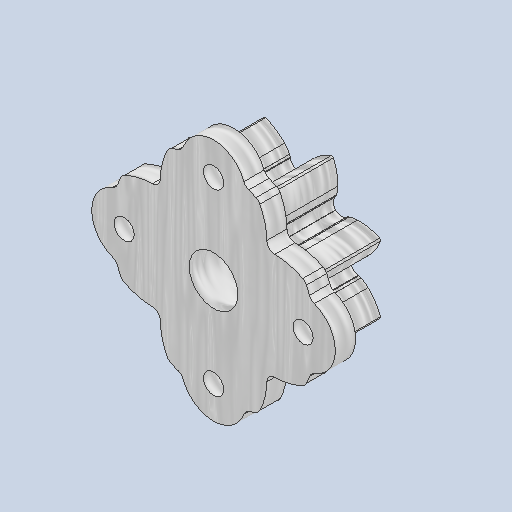
# Autodesk Inventor part: アーム 2段目ギア 小ギア 8
Saved by Autodesk Inventor 2023 (Build 270158030, 158C)
## iProperties
Created: 2020-05-02
Part Number: アーム 2段目ギア 小ギア 8
Material: アルミニウム 7075
Document SubType Name: Modeling
Designer: mozar
Density: 2.81 g/cm^3
Appearance: サテン - ブラシ仕上げ 重厚
Author: mozar
Autodesk Inventor part; units mm, degrees
ref_plane "YZ Plane" through (0, 0, 0) normal (1, 0, 0) x (0, 1, 0)
ref_plane "XZ Plane" through (0, 0, 0) normal (0, 1, 0) x (-1, 0, 0)
ref_plane "XY Plane" through (0, 0, 0) normal (0, 0, 1) x (1, 0, 0)
sketch "スケッチ1" plane through (0, 0, 0) normal (0, 0, 1) x (1, 0, 0)
  arc A0 (149.6102, 112.7227) -> (149.5189, 112.4482) centre (150.664, 112.2197) ccw
  arc A1 (150.2091, 113.6063) -> (149.6102, 112.7227) centre (152.6236, 111.3248) ccw
  arc A2 (152.5503, 115.1567) -> (150.2091, 113.6063) centre (154.7206, 109.3368) ccw
  arc A3 (143.8242, 111.2458) -> (143.9538, 110.9871) centre (144.9251, 111.6353) ccw
  arc A4 (143.623, 112.2941) -> (143.8242, 111.2458) centre (146.9435, 112.3881) ccw
  arc A5 (144.1821, 115.0459) -> (143.623, 112.2941) centre (149.832, 112.4652) ccw
  arc A6 (140.7773, 106.1102) -> (141.0518, 106.0189) centre (141.2803, 107.164) ccw
  arc A7 (139.8937, 106.7091) -> (140.7773, 106.1102) centre (142.1752, 109.1236) ccw
  arc A8 (138.3433, 109.0503) -> (139.8937, 106.7091) centre (144.1632, 111.2206) ccw
  arc A9 (142.2542, 100.3242) -> (142.5129, 100.4538) centre (141.8647, 101.4251) ccw
  arc A10 (141.2059, 100.123) -> (142.2542, 100.3242) centre (141.1119, 103.4435) ccw
  arc A11 (138.4541, 100.6821) -> (141.2059, 100.123) centre (141.0348, 106.332) ccw
  arc A12 (147.3898, 97.2773) -> (147.4811, 97.5518) centre (146.336, 97.7803) ccw
  arc A13 (146.7909, 96.3937) -> (147.3898, 97.2773) centre (144.3764, 98.6752) ccw
  arc A14 (144.4497, 94.8433) -> (146.7909, 96.3937) centre (142.2794, 100.6632) ccw
  arc A15 (153.1758, 98.7542) -> (153.0462, 99.0129) centre (152.0749, 98.3647) ccw
  arc A16 (153.377, 97.7059) -> (153.1758, 98.7542) centre (150.0565, 97.6119) ccw
  arc A17 (152.8179, 94.9541) -> (153.377, 97.7059) centre (147.168, 97.5348) ccw
  arc A18 (156.2227, 103.8898) -> (155.9482, 103.9811) centre (155.7197, 102.836) ccw
  arc A19 (157.1063, 103.2909) -> (156.2227, 103.8898) centre (154.8248, 100.8764) ccw
  arc A20 (158.6567, 100.9497) -> (157.1063, 103.2909) centre (152.8368, 98.7794) ccw
  arc A21 (154.7458, 109.6758) -> (154.4871, 109.5462) centre (155.1353, 108.5749) ccw
  arc A22 (155.7941, 109.877) -> (154.7458, 109.6758) centre (155.8881, 106.5565) ccw
  arc A23 (158.5459, 109.3179) -> (155.7941, 109.877) centre (155.9652, 103.668) ccw
  arc A24 (147.4811, 112.4482) -> (147.3898, 112.7227) centre (146.336, 112.2197) ccw
  arc A25 (147.3898, 112.7227) -> (146.7909, 113.6063) centre (144.3764, 111.3248) ccw
  arc A26 (146.7909, 113.6063) -> (144.4497, 115.1567) centre (142.2794, 109.3368) ccw
  arc A27 (142.5129, 109.5462) -> (142.2542, 109.6758) centre (141.8647, 108.5749) ccw
  arc A28 (142.2542, 109.6758) -> (141.2059, 109.877) centre (141.1119, 106.5565) ccw
  arc A29 (141.2059, 109.877) -> (138.4541, 109.3179) centre (141.0348, 103.668) ccw
  arc A30 (141.0518, 103.9811) -> (140.7773, 103.8898) centre (141.2803, 102.836) ccw
  arc A31 (140.7773, 103.8898) -> (139.8937, 103.2909) centre (142.1752, 100.8764) ccw
  arc A32 (139.8937, 103.2909) -> (138.3433, 100.9497) centre (144.1632, 98.7794) ccw
  arc A33 (143.9538, 99.0129) -> (143.8242, 98.7542) centre (144.9251, 98.3647) ccw
  arc A34 (143.8242, 98.7542) -> (143.623, 97.7059) centre (146.9435, 97.6119) ccw
  arc A35 (143.623, 97.7059) -> (144.1821, 94.9541) centre (149.832, 97.5348) ccw
  arc A36 (149.5189, 97.5518) -> (149.6102, 97.2773) centre (150.664, 97.7803) ccw
  arc A37 (149.6102, 97.2773) -> (150.2091, 96.3937) centre (152.6236, 98.6752) ccw
  arc A38 (150.2091, 96.3937) -> (152.5503, 94.8433) centre (154.7206, 100.6632) ccw
  arc A39 (154.4871, 100.4538) -> (154.7458, 100.3242) centre (155.1353, 101.4251) ccw
  arc A40 (154.7458, 100.3242) -> (155.7941, 100.123) centre (155.8881, 103.4435) ccw
  arc A41 (155.7941, 100.123) -> (158.5459, 100.6821) centre (155.9652, 106.332) ccw
  arc A42 (155.9482, 106.0189) -> (156.2227, 106.1102) centre (155.7197, 107.164) ccw
  arc A43 (156.2227, 106.1102) -> (157.1063, 106.7091) centre (154.8248, 109.1236) ccw
  arc A44 (157.1063, 106.7091) -> (158.6567, 109.0503) centre (152.8368, 111.2206) ccw
  arc A45 (153.0462, 110.9871) -> (153.1758, 111.2458) centre (152.0749, 111.6353) ccw
  arc A46 (153.1758, 111.2458) -> (153.377, 112.2941) centre (150.0565, 112.3881) ccw
  arc A47 (153.377, 112.2941) -> (152.8179, 115.0459) centre (147.168, 112.4652) ccw
  arc A48 (149.3809, 111.44) -> (147.6191, 111.44) centre (148.5, 105) ccw
  arc A49 (144.5691, 110.1767) -> (143.3233, 108.9309) centre (148.5, 105) ccw
  arc A50 (142.06, 105.8809) -> (142.06, 104.1191) centre (148.5, 105) ccw
  arc A51 (143.3233, 101.0691) -> (144.5691, 99.8233) centre (148.5, 105) ccw
  arc A52 (147.6191, 98.56) -> (149.3809, 98.56) centre (148.5, 105) ccw
  arc A53 (152.4309, 99.8233) -> (153.6767, 101.0691) centre (148.5, 105) ccw
  arc A54 (154.94, 104.1191) -> (154.94, 105.8809) centre (148.5, 105) ccw
  arc A55 (153.6767, 108.9309) -> (152.4309, 110.1767) centre (148.5, 105) ccw
  arc A56 (144.4497, 115.1567) -> (144.1821, 115.0459) centre (148.5, 105) ccw
  arc A57 (138.4541, 109.3179) -> (138.3433, 109.0503) centre (148.5, 105) ccw
  arc A58 (138.3433, 100.9497) -> (138.4541, 100.6821) centre (148.5, 105) ccw
  arc A59 (144.1821, 94.9541) -> (144.4497, 94.8433) centre (148.5, 105) ccw
  arc A60 (152.5503, 94.8433) -> (152.8179, 94.9541) centre (148.5, 105) ccw
  arc A61 (158.5459, 100.6821) -> (158.6567, 100.9497) centre (148.5, 105) ccw
  arc A62 (158.6567, 109.0503) -> (158.5459, 109.3179) centre (148.5, 105) ccw
  arc A63 (152.8179, 115.0459) -> (152.5503, 115.1567) centre (148.5, 105) ccw
  line L0 (149.3809, 111.44) -> (149.5189, 112.4482)
  line L1 (144.5691, 110.1767) -> (143.9538, 110.9871)
  line L2 (142.06, 105.8809) -> (141.0518, 106.0189)
  line L3 (143.3233, 101.0691) -> (142.5129, 100.4538)
  line L4 (147.6191, 98.56) -> (147.4811, 97.5518)
  line L5 (152.4309, 99.8233) -> (153.0462, 99.0129)
  line L6 (154.94, 104.1191) -> (155.9482, 103.9811)
  line L7 (153.6767, 108.9309) -> (154.4871, 109.5462)
  line L8 (147.6191, 111.44) -> (147.4811, 112.4482)
  line L9 (143.3233, 108.9309) -> (142.5129, 109.5462)
  line L10 (142.06, 104.1191) -> (141.0518, 103.9811)
  line L11 (144.5691, 99.8233) -> (143.9538, 99.0129)
  line L12 (149.3809, 98.56) -> (149.5189, 97.5518)
  line L13 (153.6767, 101.0691) -> (154.4871, 100.4538)
  line L14 (154.94, 105.8809) -> (155.9482, 106.0189)
  line L15 (152.4309, 110.1767) -> (153.0462, 110.9871)
  line L16 (135.5655, 105) -> (161.4345, 105)
  line L17 (148.5, 92.0655) -> (148.5, 117.9345)
  line L18 (179.4346, 115.9346) -> (249.4346, 115.9346)
  line L19 (179.4346, 107.9346) -> (249.4346, 107.9346)
  line L20 (179.4346, 99.9346) -> (249.4346, 99.9346)
  line L21 (179.4346, 91.9346) -> (249.4346, 91.9346)
  line L22 (179.4346, 83.9346) -> (249.4346, 83.9346)
  line L23 (179.4346, 75.9346) -> (249.4346, 75.9346)
  line L24 (179.4346, 67.9346) -> (249.4346, 67.9346)
  line L25 (179.4346, 59.9346) -> (249.4346, 59.9346)
  line L26 (179.4346, 51.9346) -> (249.4346, 51.9346)
  line L27 (179.4346, 43.9346) -> (249.4346, 43.9346)
  line L28 (179.4346, 35.9346) -> (249.4346, 35.9346)
  line L29 (179.4346, 27.9346) -> (249.4346, 27.9346)
  line L30 (179.4346, 19.9346) -> (249.4346, 19.9346)
  line L31 (179.4346, 115.9346) -> (179.4346, 19.9346)
  line L32 (249.4346, 115.9346) -> (249.4346, 19.9346)
  line L33 (214.4346, 107.9346) -> (214.4346, 19.9346)
  point P0 (0, 0)
  point P1 (185.4346, 109.9346)
  point P2 (187.9346, 101.9346)
  point P3 (187.9346, 93.9346)
  point P4 (185.4346, 85.9346)
  point P5 (187.9346, 77.9346)
  point P6 (182.9346, 69.9346)
  point P7 (185.4346, 61.9346)
  point P8 (185.4346, 53.9346)
  point P9 (185.4346, 45.9346)
  point P10 (187.9346, 37.9346)
  point P11 (187.9346, 29.9346)
  point P12 (185.4346, 21.9346)
  point P13 (215.4346, 101.9346)
  point P14 (231.6846, 93.9346)
  point P15 (231.6846, 85.9346)
  point P16 (227.9346, 77.9346)
  point P17 (230.4346, 69.9346)
  point P18 (224.1846, 61.9346)
  point P19 (224.1846, 53.9346)
  point P20 (230.4346, 45.9346)
  point P21 (225.4346, 37.9346)
  point P22 (232.9346, 29.9346)
  point P23 (232.9346, 21.9346)
  point P24 (149.5, 131.4345)
  point P25 (149.5, 125.4345)
  point P26 (166.75, 131.4345)
  point P27 (168.875, 125.4345)
  constraints: 128 point on circle, 64 centre point, 64 end point, 2 midpoint, 1 horizontal, 1 vertical, 268 other
extrude "押し出し1" add sketch "スケッチ1" against normal blind 8 contours A1 A2 A63 A47 A46 A45 L15 A55 L7 A21 A22 A23 A62 A44 A43 A42 L14 A54 L16 L17 A48 L0 A0 | L17 L16 A50 L2 A6 A7 A8 A57 A29 A28 A27 L9 A49 L1 A3 A4 A5 A56 A26 A25 A24 L8 A48 | L17 A52 L4 A12 A13 A14 A59 A35 A34 A33 L11 A51 L3 A9 A10 A11 A58 A32 A31 A30 L10 A50 L16 | L16 A54 L6 A18 A19 A20 A61 A41 A40 A39 L13 A53 L5 A15 A16 A17 A60 A38 A37 A36 L12 A52 L17
fillet "フィレット1" radius 1 16 edges at (142.06, 105.8809, -4) (143.3233, 108.9309, -4) (144.5691, 110.1767, -4) (147.6191, 111.44, -4) (149.3809, 111.44, -4) (152.4309, 110.1767, -4) (153.6767, 108.9309, -4) (154.94, 105.8809, -4) (154.94, 104.1191, -4) (153.6767, 101.0691, -4) (152.4309, 99.8233, -4) (149.3809, 98.56, -4) (147.6191, 98.56, -4) (144.5691, 99.8233, -4) (143.3233, 101.0691, -4) (142.06, 104.1191, -4)
sketch "スケッチ2" plane through (0, 0, 0) normal (0, 0, 1) x (1, 0, 0)
  arc A0 (153.1771, 111.2494) -> (153.1747, 111.2428) centre (154.1165, 110.9066) ccw projected
  arc A1 (153.0462, 110.9871) -> (153.1747, 111.2428) centre (152.0749, 111.6353) ccw projected
  line L0 (153.0462, 110.9871) -> (152.9951, 110.9198) projected
  arc A2 (152.9951, 110.9198) -> (153.086, 109.6064) centre (153.7915, 110.315) ccw projected
  arc A3 (153.1064, 109.586) -> (153.086, 109.6064) centre (148.5, 105) ccw projected
  arc A4 (153.1064, 109.586) -> (154.4198, 109.4951) centre (153.815, 110.2915) ccw projected
  line L1 (154.4198, 109.4951) -> (154.4871, 109.5462) projected
  arc A5 (154.7428, 109.6747) -> (154.4871, 109.5462) centre (155.1353, 108.5749) ccw projected
  arc A6 (154.7428, 109.6747) -> (154.7494, 109.6771) centre (154.4066, 110.6165) ccw projected
  arc A7 (155.7941, 109.877) -> (154.7494, 109.6771) centre (155.8881, 106.5565) ccw projected
  arc A8 (158.5459, 109.3179) -> (155.7941, 109.877) centre (155.9652, 103.668) ccw projected
  arc A9 (158.6567, 109.0503) -> (158.5459, 109.3179) centre (148.5, 105) ccw projected
  arc A10 (157.1063, 106.7091) -> (158.6567, 109.0503) centre (152.8368, 111.2206) ccw projected
  arc A11 (156.2262, 106.1118) -> (157.1063, 106.7091) centre (154.8248, 109.1236) ccw projected
  arc A12 (156.2262, 106.1118) -> (156.2198, 106.1088) centre (156.6481, 105.2052) ccw projected
  arc A13 (155.9482, 106.0189) -> (156.2198, 106.1088) centre (155.7197, 107.164) ccw projected
  line L2 (155.9482, 106.0189) -> (155.8645, 106.0074) projected
  arc A14 (155.8645, 106.0074) -> (155, 105.0144) centre (156, 105.0166) ccw projected
  arc A15 (155, 104.9856) -> (155, 105.0144) centre (148.5, 105) ccw projected
  arc A16 (155, 104.9856) -> (155.8645, 103.9926) centre (156, 104.9834) ccw projected
  line L3 (155.8645, 103.9926) -> (155.9482, 103.9811) projected
  arc A17 (156.2198, 103.8912) -> (155.9482, 103.9811) centre (155.7197, 102.836) ccw projected
  arc A18 (156.2198, 103.8912) -> (156.2262, 103.8882) centre (156.6481, 104.7948) ccw projected
  arc A19 (157.1063, 103.2909) -> (156.2262, 103.8882) centre (154.8248, 100.8764) ccw projected
  arc A20 (158.6567, 100.9497) -> (157.1063, 103.2909) centre (152.8368, 98.7794) ccw projected
  arc A21 (158.5459, 100.6821) -> (158.6567, 100.9497) centre (148.5, 105) ccw projected
  arc A22 (155.7941, 100.123) -> (158.5459, 100.6821) centre (155.9652, 106.332) ccw projected
  arc A23 (154.7494, 100.3229) -> (155.7941, 100.123) centre (155.8881, 103.4435) ccw projected
  arc A24 (154.7494, 100.3229) -> (154.7428, 100.3253) centre (154.4066, 99.3835) ccw projected
  arc A25 (154.4871, 100.4538) -> (154.7428, 100.3253) centre (155.1353, 101.4251) ccw projected
  line L4 (154.4871, 100.4538) -> (154.4198, 100.5049) projected
  arc A26 (154.4198, 100.5049) -> (153.1064, 100.414) centre (153.815, 99.7085) ccw projected
  arc A27 (153.086, 100.3936) -> (153.1064, 100.414) centre (148.5, 105) ccw projected
  arc A28 (153.086, 100.3936) -> (152.9951, 99.0802) centre (153.7915, 99.685) ccw projected
  line L5 (152.9951, 99.0802) -> (153.0462, 99.0129) projected
  arc A29 (153.1747, 98.7572) -> (153.0462, 99.0129) centre (152.0749, 98.3647) ccw projected
  arc A30 (153.1747, 98.7572) -> (153.1771, 98.7506) centre (154.1165, 99.0934) ccw projected
  arc A31 (153.377, 97.7059) -> (153.1771, 98.7506) centre (150.0565, 97.6119) ccw projected
  arc A32 (152.8179, 94.9541) -> (153.377, 97.7059) centre (147.168, 97.5348) ccw projected
  arc A33 (152.5503, 94.8433) -> (152.8179, 94.9541) centre (148.5, 105) ccw projected
  arc A34 (150.2091, 96.3937) -> (152.5503, 94.8433) centre (154.7206, 100.6632) ccw projected
  arc A35 (149.6118, 97.2738) -> (150.2091, 96.3937) centre (152.6236, 98.6752) ccw projected
  arc A36 (149.6118, 97.2738) -> (149.6088, 97.2802) centre (148.7052, 96.8519) ccw projected
  arc A37 (149.5189, 97.5518) -> (149.6088, 97.2802) centre (150.664, 97.7803) ccw projected
  line L6 (149.5189, 97.5518) -> (149.5074, 97.6355) projected
  arc A38 (149.5074, 97.6355) -> (148.5144, 98.5) centre (148.5166, 97.5) ccw projected
  arc A39 (148.4856, 98.5) -> (148.5144, 98.5) centre (148.5, 105) ccw projected
  arc A40 (148.4856, 98.5) -> (147.4926, 97.6355) centre (148.4834, 97.5) ccw projected
  line L7 (147.4926, 97.6355) -> (147.4811, 97.5518) projected
  arc A41 (147.3912, 97.2802) -> (147.4811, 97.5518) centre (146.336, 97.7803) ccw projected
  arc A42 (147.3912, 97.2802) -> (147.3882, 97.2738) centre (148.2948, 96.8519) ccw projected
  arc A43 (146.7909, 96.3937) -> (147.3882, 97.2738) centre (144.3764, 98.6752) ccw projected
  arc A44 (144.4497, 94.8433) -> (146.7909, 96.3937) centre (142.2794, 100.6632) ccw projected
  arc A45 (144.1821, 94.9541) -> (144.4497, 94.8433) centre (148.5, 105) ccw projected
  arc A46 (143.623, 97.7059) -> (144.1821, 94.9541) centre (149.832, 97.5348) ccw projected
  arc A47 (143.8229, 98.7506) -> (143.623, 97.7059) centre (146.9435, 97.6119) ccw projected
  arc A48 (143.8229, 98.7506) -> (143.8253, 98.7572) centre (142.8835, 99.0934) ccw projected
  arc A49 (143.9538, 99.0129) -> (143.8253, 98.7572) centre (144.9251, 98.3647) ccw projected
  line L8 (143.9538, 99.0129) -> (144.0049, 99.0802) projected
  arc A50 (144.0049, 99.0802) -> (143.914, 100.3936) centre (143.2085, 99.685) ccw projected
  arc A51 (143.8936, 100.414) -> (143.914, 100.3936) centre (148.5, 105) ccw projected
  arc A52 (143.8936, 100.414) -> (142.5802, 100.5049) centre (143.185, 99.7085) ccw projected
  line L9 (142.5802, 100.5049) -> (142.5129, 100.4538) projected
  arc A53 (142.2572, 100.3253) -> (142.5129, 100.4538) centre (141.8647, 101.4251) ccw projected
  arc A54 (142.2572, 100.3253) -> (142.2506, 100.3229) centre (142.5934, 99.3835) ccw projected
  arc A55 (141.2059, 100.123) -> (142.2506, 100.3229) centre (141.1119, 103.4435) ccw projected
  arc A56 (138.4541, 100.6821) -> (141.2059, 100.123) centre (141.0348, 106.332) ccw projected
  arc A57 (138.3433, 100.9497) -> (138.4541, 100.6821) centre (148.5, 105) ccw projected
  arc A58 (139.8937, 103.2909) -> (138.3433, 100.9497) centre (144.1632, 98.7794) ccw projected
  arc A59 (140.7738, 103.8882) -> (139.8937, 103.2909) centre (142.1752, 100.8764) ccw projected
  arc A60 (140.7738, 103.8882) -> (140.7802, 103.8912) centre (140.3519, 104.7948) ccw projected
  arc A61 (141.0518, 103.9811) -> (140.7802, 103.8912) centre (141.2803, 102.836) ccw projected
  line L10 (141.0518, 103.9811) -> (141.1355, 103.9926) projected
  arc A62 (141.1355, 103.9926) -> (142, 104.9856) centre (141, 104.9834) ccw projected
  arc A63 (142, 105.0144) -> (142, 104.9856) centre (148.5, 105) ccw projected
  arc A64 (142, 105.0144) -> (141.1355, 106.0074) centre (141, 105.0166) ccw projected
  line L11 (141.1355, 106.0074) -> (141.0518, 106.0189) projected
  arc A65 (140.7802, 106.1088) -> (141.0518, 106.0189) centre (141.2803, 107.164) ccw projected
  arc A66 (140.7802, 106.1088) -> (140.7738, 106.1118) centre (140.3519, 105.2052) ccw projected
  arc A67 (139.8937, 106.7091) -> (140.7738, 106.1118) centre (142.1752, 109.1236) ccw projected
  arc A68 (138.3433, 109.0503) -> (139.8937, 106.7091) centre (144.1632, 111.2206) ccw projected
  arc A69 (138.4541, 109.3179) -> (138.3433, 109.0503) centre (148.5, 105) ccw projected
  arc A70 (141.2059, 109.877) -> (138.4541, 109.3179) centre (141.0348, 103.668) ccw projected
  arc A71 (142.2506, 109.6771) -> (141.2059, 109.877) centre (141.1119, 106.5565) ccw projected
  arc A72 (142.2506, 109.6771) -> (142.2572, 109.6747) centre (142.5934, 110.6165) ccw projected
  arc A73 (142.5129, 109.5462) -> (142.2572, 109.6747) centre (141.8647, 108.5749) ccw projected
  line L12 (142.5129, 109.5462) -> (142.5802, 109.4951) projected
  arc A74 (142.5802, 109.4951) -> (143.8936, 109.586) centre (143.185, 110.2915) ccw projected
  arc A75 (143.914, 109.6064) -> (143.8936, 109.586) centre (148.5, 105) ccw projected
  arc A76 (143.914, 109.6064) -> (144.0049, 110.9198) centre (143.2085, 110.315) ccw projected
  line L13 (144.0049, 110.9198) -> (143.9538, 110.9871) projected
  arc A77 (143.8253, 111.2428) -> (143.9538, 110.9871) centre (144.9251, 111.6353) ccw projected
  arc A78 (143.8253, 111.2428) -> (143.8229, 111.2494) centre (142.8835, 110.9066) ccw projected
  arc A79 (143.623, 112.2941) -> (143.8229, 111.2494) centre (146.9435, 112.3881) ccw projected
  arc A80 (144.1821, 115.0459) -> (143.623, 112.2941) centre (149.832, 112.4652) ccw projected
  arc A81 (144.4497, 115.1567) -> (144.1821, 115.0459) centre (148.5, 105) ccw projected
  arc A82 (146.7909, 113.6063) -> (144.4497, 115.1567) centre (142.2794, 109.3368) ccw projected
  arc A83 (147.3882, 112.7262) -> (146.7909, 113.6063) centre (144.3764, 111.3248) ccw projected
  arc A84 (147.3882, 112.7262) -> (147.3912, 112.7198) centre (148.2948, 113.1481) ccw projected
  arc A85 (147.4811, 112.4482) -> (147.3912, 112.7198) centre (146.336, 112.2197) ccw projected
  line L14 (147.4811, 112.4482) -> (147.4926, 112.3645) projected
  arc A86 (147.4926, 112.3645) -> (148.4856, 111.5) centre (148.4834, 112.5) ccw projected
  arc A87 (148.5144, 111.5) -> (148.4856, 111.5) centre (148.5, 105) ccw projected
  arc A88 (148.5144, 111.5) -> (149.5074, 112.3645) centre (148.5166, 112.5) ccw projected
  line L15 (149.5074, 112.3645) -> (149.5189, 112.4482) projected
  arc A89 (149.6088, 112.7198) -> (149.5189, 112.4482) centre (150.664, 112.2197) ccw projected
  arc A90 (149.6088, 112.7198) -> (149.6118, 112.7262) centre (148.7052, 113.1481) ccw projected
  arc A91 (150.2091, 113.6063) -> (149.6118, 112.7262) centre (152.6236, 111.3248) ccw projected
  arc A92 (152.5503, 115.1567) -> (150.2091, 113.6063) centre (154.7206, 109.3368) ccw projected
  arc A93 (152.8179, 115.0459) -> (152.5503, 115.1567) centre (148.5, 105) ccw projected
  arc A94 (153.377, 112.2941) -> (152.8179, 115.0459) centre (147.168, 112.4652) ccw projected
  arc A95 (153.1771, 111.2494) -> (153.377, 112.2941) centre (150.0565, 112.3881) ccw projected
  arc A96 (148.0715, 113.4456) -> (149.5921, 109.5599) centre (150.664, 112.2197) ccw
  line L16 (149.5921, 109.5599) -> (149.16, 112.7186)
  arc A97 (149.16, 112.7186) -> (148.9285, 113.4456) centre (146.336, 112.2197) ccw
  arc A98 (148.9285, 113.4456) -> (148.0209, 114.7797) centre (144.3764, 111.3248) ccw
  arc A99 (148.0209, 114.7797) -> (144.4127, 116.9552) centre (142.2794, 109.3368) ccw
  arc A100 (144.4127, 116.9552) -> (142.9366, 116.3437) centre (148.5, 105) ccw
  arc A101 (142.9366, 116.3437) -> (141.9234, 112.2541) centre (149.832, 112.4652) ccw
  arc A102 (141.9234, 112.2541) -> (142.2251, 110.6689) centre (146.9435, 112.3881) ccw
  arc A103 (142.2251, 110.6689) -> (142.5754, 109.9912) centre (144.9251, 111.6353) ccw
  line L17 (142.5754, 109.9912) -> (144.5035, 107.4521)
  arc A104 (144.5035, 107.4521) -> (142.8311, 111.2749) centre (141.8647, 108.5749) ccw
  arc A105 (142.8311, 111.2749) -> (141.2459, 111.5766) centre (141.1119, 106.5565) ccw
  arc A106 (141.2459, 111.5766) -> (137.1563, 110.5634) centre (141.0348, 103.668) ccw
  arc A107 (137.1563, 110.5634) -> (136.5448, 109.0873) centre (148.5, 105) ccw
  arc A108 (136.5448, 109.0873) -> (138.7203, 105.4791) centre (144.1632, 111.2206) ccw
  arc A109 (138.7203, 105.4791) -> (140.0544, 104.5715) centre (142.1752, 109.1236) ccw
  arc A110 (140.0544, 104.5715) -> (143.9401, 106.0921) centre (141.2803, 107.164) ccw
  line L18 (143.9401, 106.0921) -> (140.7814, 105.66)
  arc A111 (140.7814, 105.66) -> (140.0544, 105.4285) centre (141.2803, 102.836) ccw
  arc A112 (140.0544, 105.4285) -> (138.7203, 104.5209) centre (142.1752, 100.8764) ccw
  arc A113 (138.7203, 104.5209) -> (136.5448, 100.9127) centre (144.1632, 98.7794) ccw
  arc A114 (136.5448, 100.9127) -> (137.1563, 99.4366) centre (148.5, 105) ccw
  arc A115 (137.1563, 99.4366) -> (141.2459, 98.4234) centre (141.0348, 106.332) ccw
  arc A116 (141.2459, 98.4234) -> (142.8311, 98.7251) centre (141.1119, 103.4435) ccw
  arc A117 (142.8311, 98.7251) -> (143.5088, 99.0754) centre (141.8647, 101.4251) ccw
  line L19 (143.5088, 99.0754) -> (146.0479, 101.0035)
  arc A118 (146.0479, 101.0035) -> (142.2251, 99.3311) centre (144.9251, 98.3647) ccw
  arc A119 (142.2251, 99.3311) -> (141.9234, 97.7459) centre (146.9435, 97.6119) ccw
  arc A120 (141.9234, 97.7459) -> (142.9366, 93.6563) centre (149.832, 97.5348) ccw
  arc A121 (142.9366, 93.6563) -> (144.4127, 93.0448) centre (148.5, 105) ccw
  arc A122 (144.4127, 93.0448) -> (148.0209, 95.2203) centre (142.2794, 100.6632) ccw
  arc A123 (148.0209, 95.2203) -> (148.9285, 96.5544) centre (144.3764, 98.6752) ccw
  arc A124 (148.9285, 96.5544) -> (147.4079, 100.4401) centre (146.336, 97.7803) ccw
  line L20 (147.4079, 100.4401) -> (147.84, 97.2814)
  arc A125 (147.84, 97.2814) -> (148.0715, 96.5544) centre (150.664, 97.7803) ccw
  arc A126 (148.0715, 96.5544) -> (148.9791, 95.2203) centre (152.6236, 98.6752) ccw
  arc A127 (148.9791, 95.2203) -> (152.5873, 93.0448) centre (154.7206, 100.6632) ccw
  arc A128 (152.5873, 93.0448) -> (154.0634, 93.6563) centre (148.5, 105) ccw
  arc A129 (154.0634, 93.6563) -> (155.0766, 97.7459) centre (147.168, 97.5348) ccw
  arc A130 (155.0766, 97.7459) -> (154.7749, 99.3311) centre (150.0565, 97.6119) ccw
  arc A131 (154.7749, 99.3311) -> (154.4246, 100.0088) centre (152.0749, 98.3647) ccw
  line L21 (154.4246, 100.0088) -> (152.4965, 102.5479)
  arc A132 (152.4965, 102.5479) -> (154.1689, 98.7251) centre (155.1353, 101.4251) ccw
  arc A133 (154.1689, 98.7251) -> (155.7541, 98.4234) centre (155.8881, 103.4435) ccw
  arc A134 (155.7541, 98.4234) -> (159.8437, 99.4366) centre (155.9652, 106.332) ccw
  arc A135 (159.8437, 99.4366) -> (160.4552, 100.9127) centre (148.5, 105) ccw
  arc A136 (160.4552, 100.9127) -> (158.2797, 104.5209) centre (152.8368, 98.7794) ccw
  arc A137 (158.2797, 104.5209) -> (156.9456, 105.4285) centre (154.8248, 100.8764) ccw
  arc A138 (156.9456, 105.4285) -> (153.0599, 103.9079) centre (155.7197, 102.836) ccw
  line L22 (153.0599, 103.9079) -> (156.2186, 104.34)
  arc A139 (156.2186, 104.34) -> (156.9456, 104.5715) centre (155.7197, 107.164) ccw
  arc A140 (156.9456, 104.5715) -> (158.2797, 105.4791) centre (154.8248, 109.1236) ccw
  arc A141 (158.2797, 105.4791) -> (160.4552, 109.0873) centre (152.8368, 111.2206) ccw
  arc A142 (160.4552, 109.0873) -> (159.8437, 110.5634) centre (148.5, 105) ccw
  arc A143 (159.8437, 110.5634) -> (155.7541, 111.5766) centre (155.9652, 103.668) ccw
  arc A144 (155.7541, 111.5766) -> (154.1689, 111.2749) centre (155.8881, 106.5565) ccw
  arc A145 (154.1689, 111.2749) -> (152.4965, 107.4521) centre (155.1353, 108.5749) ccw
  line L23 (152.4965, 107.4521) -> (154.4246, 109.9912)
  arc A146 (154.4246, 109.9912) -> (154.7749, 110.6689) centre (152.0749, 111.6353) ccw
  arc A147 (154.7749, 110.6689) -> (155.0766, 112.2541) centre (150.0565, 112.3881) ccw
  arc A148 (155.0766, 112.2541) -> (154.0634, 116.3437) centre (147.168, 112.4652) ccw
  arc A149 (154.0634, 116.3437) -> (152.5873, 116.9552) centre (148.5, 105) ccw
  arc A150 (152.5873, 116.9552) -> (148.9791, 114.7797) centre (154.7206, 109.3368) ccw
  arc A151 (148.9791, 114.7797) -> (148.0715, 113.4456) centre (152.6236, 111.3248) ccw
  line L24 (127.4235, 105) -> (169.5765, 105)
  line L25 (148.5, 122.1939) -> (148.5, 87.8061)
  circle A152 centre (148.5, 116.0626) radius 1.25
  circle A153 centre (148.5, 116.0626) radius 4
  circle A154 centre (137.4374, 105) radius 1.25
  circle A155 centre (159.5626, 105) radius 1.25
  circle A156 centre (148.5, 93.9374) radius 1.25
  circle A157 centre (137.4374, 105) radius 4
  circle A158 centre (159.5626, 105) radius 4
  circle A159 centre (148.5, 93.9374) radius 4
  point P0 (0, 0)
  point P1 (144.5894, 116.9035)
  point P2 (142.001, 111.499)
  point P3 (136.5965, 108.9106)
  point P4 (136.5965, 101.0894)
  point P5 (142.001, 98.501)
  point P6 (144.5894, 93.0965)
  point P7 (152.4106, 93.0965)
  point P8 (154.999, 98.501)
  point P9 (160.4035, 101.0894)
  point P10 (160.4035, 108.9106)
  point P11 (154.999, 111.499)
  point P12 (152.4106, 116.9035)
  dimension "d3" = 1.7
  dimension "d4" = 2.5
  dimension "d5" = 8
  dimension "d6" = 2.5
  dimension "d7" = 2.5
  dimension "d8" = 2.5
  dimension "d9" = 8
  dimension "d10" = 8
  dimension "d11" = 8
  constraints: 112 point on circle, 64 centre point, 20 end point, 6 coincident, 4 point on line, 4 tangent, 2 midpoint, 1 horizontal, 1 vertical, 63 other
  measures "d3" radial gap between concentric circles of A91 A151
  measures "d4" diameter of A152
  measures "d5" diameter of A153
  measures "d6" diameter of A154
  measures "d7" diameter of A155
  measures "d8" diameter of A156
  measures "d9" diameter of A157
  measures "d10" diameter of A158
  measures "d11" diameter of A159
extrude "押し出し2" add sketch "スケッチ2" along normal blind 2.5 contours A95 A94 A93 A92 A153 A150 A149 A148 A147 A144 A145 A2 L0 A1 A0 | A0 A1 L0 A2 A145 L23 A4 L1 A5 A6 A7 A8 A9 A10 A158 A14 A138 L24 L25 A96 L16 A88 A153 A92 A93 A94 A95 | A145 A144 A147 A146 L23 A4 A3 A2 | A2 A3 A4 L23 A145 | A153 A88 L15 A89 A90 A91 A92 | A92 A91 A90 A89 L15 A88 A153 L16 A97 A98 A151 A150 | A88 L16 A153 | A144 A143 A142 A141 A158 A10 A9 A8 A7 A6 A5 L1 A4 L23 A146 A147 | L16 A96 L25 A87 A88 | A88 A87 L25 A153 L16 | A153 L25 A98 A97 L16 | A150 A152 L25 A153 | A153 A96 A151 L25 | L25 A87 A86 A96 A153 | A150 A151 L25 A152 | L25 A152 A99 A153 | L25 A96 A86 A87 | L25 L24 A110 L18 A64 A157 A68 A69 A70 A71 A72 A73 L12 A74 L17 A104 A76 L13 A77 A78 A79 A80 A81 A82 A153 A86 A96 | A151 A96 A153 A86 L14 A85 A84 A83 A82 A99 A98 | A98 A99 A152 L25 | A96 A86 A153 | A153 A82 A81 A80 A79 A78 A77 L13 A76 A104 A105 A102 A101 A100 A99 | L25 A124 L20 A40 A159 A44 A45 A46 A47 A48 A49 L8 A50 L19 A118 A52 L9 A53 A54 A55 A56 A57 A58 A157 A62 A110 L24 | L24 A138 L22 A16 A158 A20 A21 A22 A23 A24 A25 L4 A26 L21 A132 A28 L5 A29 A30 A31 A32 A33 A34 A159 A38 A124 L25 | A153 A82 A83 A84 A85 L14 A86 | A158 L24 A155 A141 | A141 A140 A137 A138 A158 A14 L2 A13 A12 A11 A10 | L24 A63 A64 L18 A110 | A110 A62 A63 L24 | L24 A15 A16 L22 A138 | A138 A14 A15 L24 | L25 A39 A40 L20 A124 | A124 A38 A39 L25 | A155 L24 A140 A141 | A158 A136 A155 L24 | A10 A11 A12 A13 L2 A14 A158 | A110 A157 L24 A63 A62 | A62 A157 A110 | L24 A157 L18 A64 A63 | A138 A158 L24 A15 A14 | A14 A158 A138 | L24 A158 L22 A16 A15 | A124 A159 L25 A39 A38 | A38 A159 A124 | L25 A159 L20 A40 A39 | A155 A136 A137 L24 | A158 A20 A19 A18 A17 L3 A16 L22 A139 A140 A137 A136 | A136 A135 A134 A133 A130 A131 L21 A26 L4 A25 A24 A23 A22 A21 A20 A158 | A157 A58 A59 A60 A61 L10 A62 | A62 L10 A61 A60 A59 A58 A157 A113 A112 A109 A110 | A110 A109 L24 A157 | L18 A157 A64 | L24 A112 A111 L18 A157 | A138 A137 L24 A158 | L22 A158 A16 | L24 A140 A139 L22 A158 | A159 A34 A35 A36 A37 L6 A38 | A38 L6 A37 A36 A35 A34 A159 A127 A126 A123 A124 | A124 A123 L25 A159 | L20 A159 A40 | L25 A126 A125 L20 A159 | A105 A104 A76 A75 A74 L17 A103 A102 | A102 A103 L17 A74 L12 A73 A72 A71 A70 A69 A68 A157 A108 A107 A106 A105 | A158 A16 L3 A17 A18 A19 A20 | A58 A57 A56 A55 A54 A53 L9 A52 A118 A119 A116 A115 A114 A113 A157 | A157 L18 A111 A112 A109 A108 A68 A67 A66 A65 L11 A64 | A64 L11 A65 A66 A67 A68 A157 | L24 A154 A108 A109 | A112 A113 A154 L24 | A34 A33 A32 A31 A30 A29 L5 A28 A132 A133 A130 A129 A128 A127 A159 | A159 L20 A125 A126 A123 A122 A44 A43 A42 A41 L7 A40 | A40 L7 A41 A42 A43 A44 A159 | L25 A156 A122 A123 | A126 A127 A156 L25 | A157 L24 A154 A113 | A159 A122 A121 A120 A119 A116 A117 L19 A50 L8 A49 A48 A47 A46 A45 A44 | A104 L17 A74 A75 A76 | A157 A108 A154 L24 | A159 L25 A156 A127 | A122 A156 L25 A159 | A133 A132 A28 A27 A26 L21 A131 A130 | A132 L21 A26 A27 A28 | A119 A118 A52 A51 A50 L19 A117 A116 | A118 L19 A50 A51 A52
sketch "スケッチ3" plane through (0, 0, -8) normal (0, 0, -1) x (-1, 0, 0)
  arc A0 (-153.1747, 111.2428) -> (-153.1771, 111.2494) centre (-154.1165, 110.9066) ccw projected
  arc A1 (-153.377, 112.2941) -> (-153.1771, 111.2494) centre (-150.0565, 112.3881) ccw projected
  arc A2 (-152.8179, 115.0459) -> (-153.377, 112.2941) centre (-147.168, 112.4652) ccw projected
  arc A3 (-152.5503, 115.1567) -> (-152.8179, 115.0459) centre (-148.5, 105) ccw projected
  arc A4 (-150.2091, 113.6063) -> (-152.5503, 115.1567) centre (-154.7206, 109.3368) ccw projected
  arc A5 (-149.6118, 112.7262) -> (-150.2091, 113.6063) centre (-152.6236, 111.3248) ccw projected
  arc A6 (-149.6118, 112.7262) -> (-149.6088, 112.7198) centre (-148.7052, 113.1481) ccw projected
  arc A7 (-149.5189, 112.4482) -> (-149.6088, 112.7198) centre (-150.664, 112.2197) ccw projected
  line L0 (-149.5189, 112.4482) -> (-149.5074, 112.3645) projected
  arc A8 (-149.5074, 112.3645) -> (-148.5144, 111.5) centre (-148.5166, 112.5) ccw projected
  arc A9 (-148.4856, 111.5) -> (-148.5144, 111.5) centre (-148.5, 105) ccw projected
  arc A10 (-148.4856, 111.5) -> (-147.4926, 112.3645) centre (-148.4834, 112.5) ccw projected
  line L1 (-147.4926, 112.3645) -> (-147.4811, 112.4482) projected
  arc A11 (-147.3912, 112.7198) -> (-147.4811, 112.4482) centre (-146.336, 112.2197) ccw projected
  arc A12 (-147.3912, 112.7198) -> (-147.3882, 112.7262) centre (-148.2948, 113.1481) ccw projected
  arc A13 (-146.7909, 113.6063) -> (-147.3882, 112.7262) centre (-144.3764, 111.3248) ccw projected
  arc A14 (-144.4497, 115.1567) -> (-146.7909, 113.6063) centre (-142.2794, 109.3368) ccw projected
  arc A15 (-144.1821, 115.0459) -> (-144.4497, 115.1567) centre (-148.5, 105) ccw projected
  arc A16 (-143.623, 112.2941) -> (-144.1821, 115.0459) centre (-149.832, 112.4652) ccw projected
  arc A17 (-143.8229, 111.2494) -> (-143.623, 112.2941) centre (-146.9435, 112.3881) ccw projected
  arc A18 (-143.8229, 111.2494) -> (-143.8253, 111.2428) centre (-142.8835, 110.9066) ccw projected
  arc A19 (-143.9538, 110.9871) -> (-143.8253, 111.2428) centre (-144.9251, 111.6353) ccw projected
  line L2 (-143.9538, 110.9871) -> (-144.0049, 110.9198) projected
  arc A20 (-144.0049, 110.9198) -> (-143.914, 109.6064) centre (-143.2085, 110.315) ccw projected
  arc A21 (-143.8936, 109.586) -> (-143.914, 109.6064) centre (-148.5, 105) ccw projected
  arc A22 (-143.8936, 109.586) -> (-142.5802, 109.4951) centre (-143.185, 110.2915) ccw projected
  line L3 (-142.5802, 109.4951) -> (-142.5129, 109.5462) projected
  arc A23 (-142.2572, 109.6747) -> (-142.5129, 109.5462) centre (-141.8647, 108.5749) ccw projected
  arc A24 (-142.2572, 109.6747) -> (-142.2506, 109.6771) centre (-142.5934, 110.6165) ccw projected
  arc A25 (-141.2059, 109.877) -> (-142.2506, 109.6771) centre (-141.1119, 106.5565) ccw projected
  arc A26 (-138.4541, 109.3179) -> (-141.2059, 109.877) centre (-141.0348, 103.668) ccw projected
  arc A27 (-138.3433, 109.0503) -> (-138.4541, 109.3179) centre (-148.5, 105) ccw projected
  arc A28 (-139.8937, 106.7091) -> (-138.3433, 109.0503) centre (-144.1632, 111.2206) ccw projected
  arc A29 (-140.7738, 106.1118) -> (-139.8937, 106.7091) centre (-142.1752, 109.1236) ccw projected
  arc A30 (-140.7738, 106.1118) -> (-140.7802, 106.1088) centre (-140.3519, 105.2052) ccw projected
  arc A31 (-141.0518, 106.0189) -> (-140.7802, 106.1088) centre (-141.2803, 107.164) ccw projected
  line L4 (-141.0518, 106.0189) -> (-141.1355, 106.0074) projected
  arc A32 (-141.1355, 106.0074) -> (-142, 105.0144) centre (-141, 105.0166) ccw projected
  arc A33 (-142, 104.9856) -> (-142, 105.0144) centre (-148.5, 105) ccw projected
  arc A34 (-142, 104.9856) -> (-141.1355, 103.9926) centre (-141, 104.9834) ccw projected
  line L5 (-141.1355, 103.9926) -> (-141.0518, 103.9811) projected
  arc A35 (-140.7802, 103.8912) -> (-141.0518, 103.9811) centre (-141.2803, 102.836) ccw projected
  arc A36 (-140.7802, 103.8912) -> (-140.7738, 103.8882) centre (-140.3519, 104.7948) ccw projected
  arc A37 (-139.8937, 103.2909) -> (-140.7738, 103.8882) centre (-142.1752, 100.8764) ccw projected
  arc A38 (-138.3433, 100.9497) -> (-139.8937, 103.2909) centre (-144.1632, 98.7794) ccw projected
  arc A39 (-138.4541, 100.6821) -> (-138.3433, 100.9497) centre (-148.5, 105) ccw projected
  arc A40 (-141.2059, 100.123) -> (-138.4541, 100.6821) centre (-141.0348, 106.332) ccw projected
  arc A41 (-142.2506, 100.3229) -> (-141.2059, 100.123) centre (-141.1119, 103.4435) ccw projected
  arc A42 (-142.2506, 100.3229) -> (-142.2572, 100.3253) centre (-142.5934, 99.3835) ccw projected
  arc A43 (-142.5129, 100.4538) -> (-142.2572, 100.3253) centre (-141.8647, 101.4251) ccw projected
  line L6 (-142.5129, 100.4538) -> (-142.5802, 100.5049) projected
  arc A44 (-142.5802, 100.5049) -> (-143.8936, 100.414) centre (-143.185, 99.7085) ccw projected
  arc A45 (-143.914, 100.3936) -> (-143.8936, 100.414) centre (-148.5, 105) ccw projected
  arc A46 (-143.914, 100.3936) -> (-144.0049, 99.0802) centre (-143.2085, 99.685) ccw projected
  line L7 (-144.0049, 99.0802) -> (-143.9538, 99.0129) projected
  arc A47 (-143.8253, 98.7572) -> (-143.9538, 99.0129) centre (-144.9251, 98.3647) ccw projected
  arc A48 (-143.8253, 98.7572) -> (-143.8229, 98.7506) centre (-142.8835, 99.0934) ccw projected
  arc A49 (-143.623, 97.7059) -> (-143.8229, 98.7506) centre (-146.9435, 97.6119) ccw projected
  arc A50 (-144.1821, 94.9541) -> (-143.623, 97.7059) centre (-149.832, 97.5348) ccw projected
  arc A51 (-144.4497, 94.8433) -> (-144.1821, 94.9541) centre (-148.5, 105) ccw projected
  arc A52 (-146.7909, 96.3937) -> (-144.4497, 94.8433) centre (-142.2794, 100.6632) ccw projected
  arc A53 (-147.3882, 97.2738) -> (-146.7909, 96.3937) centre (-144.3764, 98.6752) ccw projected
  arc A54 (-147.3882, 97.2738) -> (-147.3912, 97.2802) centre (-148.2948, 96.8519) ccw projected
  arc A55 (-147.4811, 97.5518) -> (-147.3912, 97.2802) centre (-146.336, 97.7803) ccw projected
  line L8 (-147.4811, 97.5518) -> (-147.4926, 97.6355) projected
  arc A56 (-147.4926, 97.6355) -> (-148.4856, 98.5) centre (-148.4834, 97.5) ccw projected
  arc A57 (-148.5144, 98.5) -> (-148.4856, 98.5) centre (-148.5, 105) ccw projected
  arc A58 (-148.5144, 98.5) -> (-149.5074, 97.6355) centre (-148.5166, 97.5) ccw projected
  line L9 (-149.5074, 97.6355) -> (-149.5189, 97.5518) projected
  arc A59 (-149.6088, 97.2802) -> (-149.5189, 97.5518) centre (-150.664, 97.7803) ccw projected
  arc A60 (-149.6088, 97.2802) -> (-149.6118, 97.2738) centre (-148.7052, 96.8519) ccw projected
  arc A61 (-150.2091, 96.3937) -> (-149.6118, 97.2738) centre (-152.6236, 98.6752) ccw projected
  arc A62 (-152.5503, 94.8433) -> (-150.2091, 96.3937) centre (-154.7206, 100.6632) ccw projected
  arc A63 (-152.8179, 94.9541) -> (-152.5503, 94.8433) centre (-148.5, 105) ccw projected
  arc A64 (-153.377, 97.7059) -> (-152.8179, 94.9541) centre (-147.168, 97.5348) ccw projected
  arc A65 (-153.1771, 98.7506) -> (-153.377, 97.7059) centre (-150.0565, 97.6119) ccw projected
  arc A66 (-153.1771, 98.7506) -> (-153.1747, 98.7572) centre (-154.1165, 99.0934) ccw projected
  arc A67 (-153.0462, 99.0129) -> (-153.1747, 98.7572) centre (-152.0749, 98.3647) ccw projected
  line L10 (-153.0462, 99.0129) -> (-152.9951, 99.0802) projected
  arc A68 (-152.9951, 99.0802) -> (-153.086, 100.3936) centre (-153.7915, 99.685) ccw projected
  arc A69 (-153.1064, 100.414) -> (-153.086, 100.3936) centre (-148.5, 105) ccw projected
  arc A70 (-153.1064, 100.414) -> (-154.4198, 100.5049) centre (-153.815, 99.7085) ccw projected
  line L11 (-154.4198, 100.5049) -> (-154.4871, 100.4538) projected
  arc A71 (-154.7428, 100.3253) -> (-154.4871, 100.4538) centre (-155.1353, 101.4251) ccw projected
  arc A72 (-154.7428, 100.3253) -> (-154.7494, 100.3229) centre (-154.4066, 99.3835) ccw projected
  arc A73 (-155.7941, 100.123) -> (-154.7494, 100.3229) centre (-155.8881, 103.4435) ccw projected
  arc A74 (-158.5459, 100.6821) -> (-155.7941, 100.123) centre (-155.9652, 106.332) ccw projected
  arc A75 (-158.6567, 100.9497) -> (-158.5459, 100.6821) centre (-148.5, 105) ccw projected
  arc A76 (-157.1063, 103.2909) -> (-158.6567, 100.9497) centre (-152.8368, 98.7794) ccw projected
  arc A77 (-156.2262, 103.8882) -> (-157.1063, 103.2909) centre (-154.8248, 100.8764) ccw projected
  arc A78 (-156.2262, 103.8882) -> (-156.2198, 103.8912) centre (-156.6481, 104.7948) ccw projected
  arc A79 (-155.9482, 103.9811) -> (-156.2198, 103.8912) centre (-155.7197, 102.836) ccw projected
  line L12 (-155.9482, 103.9811) -> (-155.8645, 103.9926) projected
  arc A80 (-155.8645, 103.9926) -> (-155, 104.9856) centre (-156, 104.9834) ccw projected
  arc A81 (-155, 105.0144) -> (-155, 104.9856) centre (-148.5, 105) ccw projected
  arc A82 (-155, 105.0144) -> (-155.8645, 106.0074) centre (-156, 105.0166) ccw projected
  line L13 (-155.8645, 106.0074) -> (-155.9482, 106.0189) projected
  arc A83 (-156.2198, 106.1088) -> (-155.9482, 106.0189) centre (-155.7197, 107.164) ccw projected
  arc A84 (-156.2198, 106.1088) -> (-156.2262, 106.1118) centre (-156.6481, 105.2052) ccw projected
  arc A85 (-157.1063, 106.7091) -> (-156.2262, 106.1118) centre (-154.8248, 109.1236) ccw projected
  arc A86 (-158.6567, 109.0503) -> (-157.1063, 106.7091) centre (-152.8368, 111.2206) ccw projected
  arc A87 (-158.5459, 109.3179) -> (-158.6567, 109.0503) centre (-148.5, 105) ccw projected
  arc A88 (-155.7941, 109.877) -> (-158.5459, 109.3179) centre (-155.9652, 103.668) ccw projected
  arc A89 (-154.7494, 109.6771) -> (-155.7941, 109.877) centre (-155.8881, 106.5565) ccw projected
  arc A90 (-154.7494, 109.6771) -> (-154.7428, 109.6747) centre (-154.4066, 110.6165) ccw projected
  arc A91 (-154.4871, 109.5462) -> (-154.7428, 109.6747) centre (-155.1353, 108.5749) ccw projected
  line L14 (-154.4871, 109.5462) -> (-154.4198, 109.4951) projected
  arc A92 (-154.4198, 109.4951) -> (-153.1064, 109.586) centre (-153.815, 110.2915) ccw projected
  arc A93 (-153.086, 109.6064) -> (-153.1064, 109.586) centre (-148.5, 105) ccw projected
  arc A94 (-153.086, 109.6064) -> (-152.9951, 110.9198) centre (-153.7915, 110.315) ccw projected
  line L15 (-152.9951, 110.9198) -> (-153.0462, 110.9871) projected
  arc A95 (-153.1747, 111.2428) -> (-153.0462, 110.9871) centre (-152.0749, 111.6353) ccw projected
  point P0 (0, 0)
hole "穴1" at (148.5, 105, -8) direction (0, 0, 1) diameter 6 depth 12 tip angle 118
fillet "フィレット2" radius 1 12 edges at (142.001, 111.499, 1.25) (136.5965, 101.0894, 1.25) (142.001, 98.501, 1.25) (144.5894, 93.0965, 1.25) (152.4106, 116.9035, 1.25) (154.999, 111.499, 1.25) (160.4035, 101.0894, 1.25) (154.999, 98.501, 1.25) (152.4106, 93.0965, 1.25) (144.5894, 116.9035, 1.25) (136.5965, 108.9106, 1.25) (160.4035, 108.9106, 1.25)
fillet "フィレット3" radius 1 16 edges at (144.4127, 93.0448, 1.25) (152.5873, 93.0448, 1.25) (154.0634, 93.6563, 1.25) (159.8437, 99.4366, 1.25) (160.4552, 100.9127, 1.25) (142.9366, 93.6563, 1.25) (137.1563, 99.4366, 1.25) (136.5448, 100.9127, 1.25) (136.5448, 109.0873, 1.25) (137.1563, 110.5634, 1.25) (142.9366, 116.3437, 1.25) (152.5873, 116.9552, 1.25) (154.0634, 116.3437, 1.25) (159.8437, 110.5634, 1.25) (160.4552, 109.0873, 1.25) (144.4127, 116.9552, 1.25)
sketch "スケッチ4" plane through (0, 0, 2.5) normal (0, 0, 1) x (1, 0, 0)
  arc A0 (152.8433, 93.1355) -> (152.2497, 92.5446) centre (153.1871, 92.1964) ccw projected
  arc A1 (144.7503, 92.5446) -> (152.2497, 92.5446) centre (148.5, 93.9374) ccw projected
  arc A2 (144.7503, 92.5446) -> (144.1567, 93.1355) centre (143.8129, 92.1964) ccw projected
  arc A3 (143.2473, 93.5091) -> (144.1567, 93.1355) centre (148.5, 105) ccw projected
  arc A4 (142.7704, 93.9677) -> (143.2473, 93.5091) centre (143.663, 94.4186) ccw projected
  arc A5 (141.9213, 97.4341) -> (142.7704, 93.9677) centre (149.832, 97.5348) ccw projected
  arc A6 (141.9213, 97.4341) -> (140.9341, 98.4213) centre (140.9213, 97.4213) ccw projected
  arc A7 (137.4677, 99.2704) -> (140.9341, 98.4213) centre (141.0348, 106.332) ccw projected
  arc A8 (137.0091, 99.7473) -> (137.4677, 99.2704) centre (137.9186, 100.163) ccw projected
  arc A9 (136.6355, 100.6567) -> (137.0091, 99.7473) centre (148.5, 105) ccw projected
  arc A10 (136.6355, 100.6567) -> (136.0446, 101.2503) centre (135.6964, 100.3129) ccw projected
  arc A11 (136.0446, 108.7497) -> (136.0446, 101.2503) centre (137.4374, 105) ccw projected
  arc A12 (136.0446, 108.7497) -> (136.6355, 109.3433) centre (135.6964, 109.6871) ccw projected
  arc A13 (137.0091, 110.2527) -> (136.6355, 109.3433) centre (148.5, 105) ccw projected
  arc A14 (137.4677, 110.7296) -> (137.0091, 110.2527) centre (137.9186, 109.837) ccw projected
  arc A15 (140.9341, 111.5787) -> (137.4677, 110.7296) centre (141.0348, 103.668) ccw projected
  arc A16 (140.9341, 111.5787) -> (141.9213, 112.5659) centre (140.9213, 112.5787) ccw projected
  arc A17 (142.7704, 116.0323) -> (141.9213, 112.5659) centre (149.832, 112.4652) ccw projected
  arc A18 (143.2473, 116.4909) -> (142.7704, 116.0323) centre (143.663, 115.5814) ccw projected
  arc A19 (144.1567, 116.8645) -> (143.2473, 116.4909) centre (148.5, 105) ccw projected
  arc A20 (144.1567, 116.8645) -> (144.7503, 117.4554) centre (143.8129, 117.8036) ccw projected
  arc A21 (152.2497, 117.4554) -> (144.7503, 117.4554) centre (148.5, 116.0626) ccw projected
  arc A22 (152.2497, 117.4554) -> (152.8433, 116.8645) centre (153.1871, 117.8036) ccw projected
  arc A23 (153.7527, 116.4909) -> (152.8433, 116.8645) centre (148.5, 105) ccw projected
  arc A24 (154.2296, 116.0323) -> (153.7527, 116.4909) centre (153.337, 115.5814) ccw projected
  arc A25 (155.0787, 112.5659) -> (154.2296, 116.0323) centre (147.168, 112.4652) ccw projected
  arc A26 (155.0787, 112.5659) -> (156.0659, 111.5787) centre (156.0787, 112.5787) ccw projected
  arc A27 (159.5323, 110.7296) -> (156.0659, 111.5787) centre (155.9652, 103.668) ccw projected
  arc A28 (159.9909, 110.2527) -> (159.5323, 110.7296) centre (159.0814, 109.837) ccw projected
  arc A29 (160.3645, 109.3433) -> (159.9909, 110.2527) centre (148.5, 105) ccw projected
  arc A30 (160.3645, 109.3433) -> (160.9554, 108.7497) centre (161.3036, 109.6871) ccw projected
  arc A31 (160.9554, 101.2503) -> (160.9554, 108.7497) centre (159.5626, 105) ccw projected
  arc A32 (160.9554, 101.2503) -> (160.3645, 100.6567) centre (161.3036, 100.3129) ccw projected
  arc A33 (159.9909, 99.7473) -> (160.3645, 100.6567) centre (148.5, 105) ccw projected
  arc A34 (159.5323, 99.2704) -> (159.9909, 99.7473) centre (159.0814, 100.163) ccw projected
  arc A35 (156.0659, 98.4213) -> (159.5323, 99.2704) centre (155.9652, 106.332) ccw projected
  arc A36 (156.0659, 98.4213) -> (155.0787, 97.4341) centre (156.0787, 97.4213) ccw projected
  arc A37 (154.2296, 93.9677) -> (155.0787, 97.4341) centre (147.168, 97.5348) ccw projected
  arc A38 (153.7527, 93.5091) -> (154.2296, 93.9677) centre (153.337, 94.4186) ccw projected
  arc A39 (152.8433, 93.1355) -> (153.7527, 93.5091) centre (148.5, 105) ccw projected
  circle A40 centre (148.5, 105) radius 3 projected
  circle A41 centre (148.5, 116.0626) radius 1.25 projected
  circle A42 centre (137.4374, 105) radius 1.25 projected
  circle A43 centre (159.5626, 105) radius 1.25 projected
  circle A44 centre (148.5, 93.9374) radius 1.25 projected
  point P0 (0, 0)
